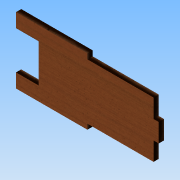
# Autodesk Inventor part: bottom2
Saved by Autodesk Inventor 2015 (Build 190159000, 159)
## iProperties
Created: 2015-12-28
Part Number: bottom2
Material: Générique
Document SubType Name: Modeling
Designer: Gregwar
Density: 1 g/cm^3
Appearance: Par défaut
Author: Gregwar
Autodesk Inventor part; units mm, degrees
ref_plane "YZ Plane" through (0, 0, 0) normal (1, 0, 0) x (0, 1, 0)
ref_plane "XZ Plane" through (0, 0, 0) normal (0, 1, 0) x (-1, 0, 0)
ref_plane "XY Plane" through (0, 0, 0) normal (0, 0, 1) x (1, 0, 0)
sketch "Esquisse1" plane through (0, 0, 0) normal (0, 1, 0) x (-1, 0, 0)
  line L0 (0, 0) -> (76, 0)
  line L1 (76, 0) -> (76, -32)
  line L2 (76, -32) -> (0, -32)
  line L3 (0, -32) -> (0, 0)
  dimension "d0" = 32
  dimension "d1" = 76
  constraints: 8 end point, 2 parallel, 1 horizontal, 1 perpendicular
  measures "d0" distance of L2.end L0.start
  measures "d1" distance of L0.start L0.end
extrude "Extrusion1" add sketch "Esquisse1" along normal blind 3
sketch "Esquisse2" plane through (0, 3, 0) normal (0, 1, 0) x (1, 0, 0)
  line L0 (-76, 0) -> (0, 0) projected
  line L1 (0, 0) -> (0, 32) projected
  line L2 (0, 32) -> (-76, 32) projected
  line L3 (-76, 32) -> (-76, 0) projected
  line L4 (-76, 0) -> (-79, 0)
  line L5 (-79, 0) -> (-79, 10.6667)
  line L6 (-79, 10.6667) -> (-76, 10.6667)
  line L7 (-76, 10.6667) -> (-76, 0)
  line L8 (-76, 16) -> (-93.4879, 16) construction
  line L9 (-76, 32) -> (0, 32)
  line L10 (-76, 0) -> (-76, 32)
  line L11 (-76, 32) -> (-79, 32)
  line L12 (-79, 32) -> (-79, 21.3333)
  line L13 (-79, 21.3333) -> (-76, 21.3333)
  line L14 (-76, 21.3333) -> (-76, 32)
  line L15 (-76, 0) -> (-38, 0)
  line L16 (-38, 0) -> (-38, -3)
  line L17 (-38, -3) -> (-76, -3)
  line L18 (-76, -3) -> (-76, 0)
  line L19 (-76, 32) -> (-38, 32)
  line L20 (-38, 32) -> (-38, 35)
  line L21 (-38, 35) -> (-76, 35)
  line L22 (-76, 35) -> (-76, 32)
  line L23 (-76, 0) -> (-79, 0)
  line L24 (-79, 0) -> (-79, -3)
  line L25 (-79, -3) -> (-76, -3)
  line L26 (-76, -3) -> (-76, 0)
  line L27 (-76, 32) -> (-79, 32)
  line L28 (-79, 32) -> (-79, 35)
  line L29 (-79, 35) -> (-76, 35)
  line L30 (-76, 35) -> (-76, 32)
  dimension "d4" = 32
  dimension "d5" = 3
  dimension "d6" = 10.6667
  dimension "d9" = 76
  dimension "d10" = 38
  dimension "d11" = 3
  constraints: 54 end point, 10 symmetric about line, 8 parallel, 5 horizontal, 4 perpendicular, 2 point on line, 1 midpoint
  measures "d4" distance of L2.end L0.start
  measures "d5" distance of L0.start L4.end
  measures "d6" distance of L4.end L5.end
  measures "d9" distance of L0.start L0.end
  measures "d10" distance of L16.end L17.end
  measures "d11" distance of L17.end L10.start
extrude "Extrusion2" add sketch "Esquisse2" against normal blind 3 contours L0 L16 L17 L18 | L22 L21 L20 L2
sketch "Esquisse6" plane through (0, 0, 0) normal (0, -1, 0) x (1, 0, 0)
  line L0 (0, 0) -> (-38, 0) projected
  line L1 (-38, 0) -> (-38, 3) projected
  line L2 (-38, 3) -> (-76, 3) projected
  line L3 (-76, -35) -> (-38, -35) projected
  line L4 (-38, -35) -> (-38, -32) projected
  line L5 (-38, -32) -> (0, -32) projected
  line L6 (0, -32) -> (0, 0) projected
  line L7 (3, -10.6667) -> (0, -10.6667)
  line L8 (0, -10.6667) -> (0, -21.3333)
  line L9 (0, -21.3333) -> (3, -21.3333)
  line L10 (3, -21.3333) -> (3, -10.6667)
  line L11 (-76, 3) -> (-76, -35) projected
  point P0 (0, -16)
  dimension "d19" = 3
  dimension "d20" = 32
  dimension "d21" = 10.6667
  constraints: 8 end point, 2 midpoint, 2 parallel, 1 horizontal, 1 perpendicular
  measures "d19" distance of L7.start L7.end
  measures "d20" distance of L5.end L0.start
  measures "d21" distance of L9.end L7.start
extrude "Extrusion5" add sketch "Esquisse6" against normal blind 3 contours L7 L10 L9 L6
sketch "Esquisse7" plane through (0, 0, 0) normal (0, -1, 0) x (1, 0, 0)
  line L0 (0, 0) -> (-38, 0) projected
  line L1 (-38, 0) -> (-38, 3) projected
  line L2 (-38, 3) -> (-76, 3) projected
  line L3 (-76, -35) -> (-38, -35) projected
  line L4 (-38, -35) -> (-38, -32) projected
  line L5 (-38, -32) -> (0, -32) projected
  line L6 (0, -32) -> (0, -21.3333) projected
  line L7 (0, -21.3333) -> (3, -21.3333) projected
  line L8 (3, -21.3333) -> (3, -10.6667) projected
  line L9 (3, -10.6667) -> (0, -10.6667) projected
  line L10 (0, -10.6667) -> (0, 0) projected
  line L11 (-76, 0) -> (-79, 0)
  line L12 (-79, 0) -> (-79, 3)
  line L13 (-79, 3) -> (-76, 3)
  line L14 (-76, 3) -> (-76, 0)
  line L15 (-76, -32) -> (-79, -32)
  line L16 (-79, -32) -> (-79, -35)
  line L17 (-79, -35) -> (-76, -35)
  line L18 (-76, -35) -> (-76, -32)
  line L19 (-76, 3) -> (-76, -35) projected
  constraints: 16 end point, 4 parallel, 2 horizontal, 2 perpendicular
extrude "Extrusion6" add sketch "Esquisse7" against normal blind 3 contours L14 L11 L12 L13 | L18 L17 L16 L15
sketch "Esquisse8" plane through (0, 0, 0) normal (0, -1, 0) x (1, 0, 0)
  line L0 (0, 0) -> (-38, 0) projected
  line L1 (-38, 0) -> (-38, 3) projected
  line L2 (-38, 3) -> (-79, 3) projected
  line L3 (-79, 3) -> (-79, 0) projected
  line L4 (-79, 0) -> (-76, 0) projected
  line L5 (-76, 0) -> (-76, -32) projected
  line L6 (-76, -32) -> (-79, -32) projected
  line L7 (-79, -32) -> (-79, -35) projected
  line L8 (-79, -35) -> (-38, -35) projected
  line L9 (-38, -35) -> (-38, -32) projected
  line L10 (-38, -32) -> (0, -32) projected
  line L11 (0, -32) -> (0, -21.3333) projected
  line L12 (0, -21.3333) -> (3, -21.3333) projected
  line L13 (3, -21.3333) -> (3, -10.6667) projected
  line L14 (3, -10.6667) -> (0, -10.6667) projected
  line L15 (0, -10.6667) -> (0, 0) projected
  line L16 (-76, 0) -> (-76, -32) projected
  line L17 (-76, -5) -> (-66, -5)
  line L18 (-66, -5) -> (-66, -27)
  line L19 (-66, -27) -> (-76, -27)
  line L20 (-76, -27) -> (-76, -5)
  line L21 (-76, -16) -> (-66, -16) construction
  line L22 (-76, -16) -> (3, -16) construction
  line L23 (3, -10.6667) -> (3, -21.3333) construction
  dimension "d26" = 10
  dimension "d27" = 22
  constraints: 12 end point, 4 midpoint, 2 parallel, 1 collinear, 1 horizontal, 1 perpendicular, 1 point on line
  measures "d26" distance of L17.start L17.end
  measures "d27" distance of L17.end L18.end
extrude "Extrusion7" cut sketch "Esquisse8" against normal through all contours L17 L18 L19 L5
sketch "Esquisse9" plane through (0, 0, 0) normal (0, -1, 0) x (1, 0, 0)
  line L0 (-66, -27) -> (-76, -27) projected
  line L1 (-76, -27) -> (-76, -32) projected
  line L2 (-76, -32) -> (-79, -32) projected
  line L3 (-79, -32) -> (-79, -35) projected
  line L4 (-79, -35) -> (-38, -35) projected
  line L5 (-38, -35) -> (-38, -32) projected
  line L6 (-38, -32) -> (0, -32) projected
  line L7 (0, -32) -> (0, -21.3333) projected
  line L8 (0, -21.3333) -> (3, -21.3333) projected
  line L9 (3, -21.3333) -> (3, -10.6667) projected
  line L10 (3, -10.6667) -> (0, -10.6667) projected
  line L11 (0, -10.6667) -> (0, 0) projected
  line L12 (0, 0) -> (-38, 0) projected
  line L13 (-38, 0) -> (-38, 3) projected
  line L14 (-38, 3) -> (-79, 3) projected
  line L15 (-79, 3) -> (-79, 0) projected
  line L16 (-79, 0) -> (-76, 0) projected
  line L17 (-76, 0) -> (-76, -5) projected
  line L18 (-76, -5) -> (-66, -5) projected
  line L19 (-66, -5) -> (-66, -27) projected
  line L20 (-76, 0) -> (-79, 0)
  line L21 (-79, 0) -> (-79, -5)
  line L22 (-79, -5) -> (-76, -5)
  line L23 (-76, -5) -> (-76, 0)
  line L24 (-76, -32) -> (-79, -32)
  line L25 (-79, -32) -> (-79, -27)
  line L26 (-79, -27) -> (-76, -27)
  line L27 (-76, -27) -> (-76, -32)
  constraints: 16 end point, 4 parallel, 2 horizontal, 2 perpendicular
extrude "Extrusion8" add sketch "Esquisse9" against normal blind 3 contours L1 L2 L25 L26 | L22 L21 L16 L17
equation "\"d6\" = 0.333333 * d4"
equation "\"d10\" = 0.5 * d9"
equation "\"d21\" = 0.333333 * d20"
